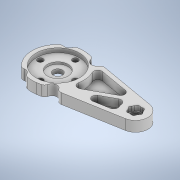
# Autodesk Inventor part: Ankle_side_pitch_frame
Saved by Autodesk Inventor 2020 (Build 240168000, 168)
## iProperties
Created: 2021-10-01
Part Number: Ankle_side_pitch_frame
Material: アルミニウム 2014-T4
Document SubType Name: Modeling
Designer: Masato Kubotera
Density: 2.8 g/cm^3
Appearance: 滑らか - 淡い灰色
Description: A2017 T5
Author: Masato Kubotera
Autodesk Inventor part; units mm, degrees
ref_plane "YZ Plane" through (0, 0, 0) normal (1, 0, 0) x (0, 1, 0)
ref_plane "XZ Plane" through (0, 0, 0) normal (0, 1, 0) x (-1, 0, 0)
ref_plane "XY Plane" through (0, 0, 0) normal (0, 0, 1) x (1, 0, 0)
sketch "スケッチ1" plane through (0, 0, 0) normal (0, 0, 1) x (1, 0, 0)
  circle A0 centre (0, 0) radius 10.5 construction
  circle A1 centre (0, 0) radius 5 construction
  circle A2 centre (0, 0) radius 5.01
  circle A3 centre (0, 0) radius 10.51
  arc A4 (2.1531, 12.3132) -> (2.1531, -12.3132) centre (0, 0) ccw
  circle A5 centre (37.7359, 0) radius 2.25
  arc A6 (38.7694, -5.9103) -> (38.7694, 5.9103) centre (37.7359, 0) ccw
  circle A7 centre (8.5, 0) radius 1.35
  circle A8 centre (0, 8.5) radius 1.35
  circle A9 centre (-8.5, 0) radius 1.35
  circle A10 centre (0, -8.5) radius 1.35
  line L0 (2.1531, 12.3132) -> (38.7694, 5.9103)
  line L1 (2.1531, -12.3132) -> (38.7694, -5.9103)
  line L2 (13.3804, 8.3196) -> (26.7879, 5.9751)
  line L3 (30.7947, -5.2745) -> (23.5904, -6.5342)
  arc A11 (2.1531, -12.3132) -> (-4.7001, 11.5827) centre (0, 0) ccw construction
  arc A12 (38.7694, 5.9103) -> (32.2717, -2.4783) centre (37.7359, 0) ccw construction
  line L4 (34.0196, 4.7105) -> (8.4896, -9.1748) construction
  line L5 (27.399, 2.248) -> (15.2168, -4.3777)
  line L6 (28.8431, 0.7568) -> (22.2903, -2.8072)
  line L7 (32.4358, 4.9875) -> (34.0196, 4.7105) construction
  line L8 (11.5743, -8.6354) -> (8.4896, -9.1748) construction
  arc A13 (31.783, -0.7501) -> (32.2717, -2.4783) centre (37.7359, 0) ccw
  arc A14 (12.2941, -2.2592) -> (11.2378, 5.4737) centre (0, 0) ccw
  line L9 (40.9229, 0) -> (40.3979, -0.9093) construction
  line L10 (39.3294, -2.76) -> (38.2794, -2.76) construction
  line L11 (36.1424, -2.76) -> (35.6174, -1.8507) construction
  line L12 (34.549, 0) -> (35.074, 0.9093) construction
  line L13 (36.1424, 2.76) -> (37.1924, 2.76) construction
  line L14 (39.3294, 2.76) -> (39.8544, 1.8507)
  arc A15 (40.3979, -0.9093) -> (40.3979, 0.9093) centre (39.8729, 0) ccw
  arc A16 (39.8544, 1.8507) -> (38.2794, 2.76) centre (38.8044, 1.8507) ccw
  arc A17 (37.1924, 2.76) -> (35.6174, 1.8507) centre (36.6674, 1.8507) ccw
  arc A18 (35.074, 0.9093) -> (35.074, -0.9093) centre (35.599, 0) ccw
  arc A19 (35.6174, -1.8507) -> (37.1924, -2.76) centre (36.6674, -1.8507) ccw
  arc A20 (38.2794, -2.76) -> (39.8544, -1.8507) centre (38.8044, -1.8507) ccw
  line L15 (40.3979, -0.9093) -> (39.8544, -1.8507)
  line L16 (39.8544, -1.8507) -> (39.3294, -2.76) construction
  line L17 (38.2794, -2.76) -> (37.1924, -2.76)
  line L18 (37.1924, -2.76) -> (36.1424, -2.76) construction
  line L19 (35.6174, -1.8507) -> (35.074, -0.9093)
  line L20 (35.074, -0.9093) -> (34.549, 0) construction
  line L21 (35.6174, 1.8507) -> (36.1424, 2.76) construction
  line L22 (35.074, 0.9093) -> (35.6174, 1.8507)
  line L23 (37.1924, 2.76) -> (38.2794, 2.76)
  line L24 (38.2794, 2.76) -> (39.3294, 2.76) construction
  line L25 (39.8544, 1.8507) -> (40.3979, 0.9093)
  line L26 (40.3979, 0.9093) -> (40.9229, 0) construction
  circle A21 centre (37.7359, 0) radius 1.55
  circle A22 centre (0, 0) radius 2.25
  line L27 (0, 0) -> (27.1359, -16.96) construction
  line L28 (37.7359, 0) -> (27.1359, -16.96) construction
  line L29 (0, 0) -> (37.7359, 0) construction
  line L30 (0, 0) -> (0.848, -0.53)
  line L31 (8.003, 10.918) -> (-6.307, -11.978) construction
  arc A23 (-3.808, -11.9058) -> (-7.6616, -9.8768) centre (-6.307, -11.978) ccw
  arc A24 (5.6301, 11.7052) -> (10.5021, 10.8532) centre (8.003, 10.918) ccw
  arc A25 (13.3804, 8.3196) -> (11.2378, 5.4737) centre (13.0359, 6.3495) ccw
  arc A26 (12.2941, -2.2592) -> (15.2168, -4.3777) centre (14.2612, -2.6207) ccw
  arc A27 (22.2903, -2.8072) -> (23.5904, -6.5342) centre (23.2459, -4.5641) ccw
  arc A28 (30.7947, -5.2745) -> (32.2717, -2.4783) centre (30.4502, -3.3043) ccw
  arc A29 (31.783, -0.7501) -> (28.8431, 0.7568) centre (29.7987, -1.0002) ccw
  arc A30 (27.399, 2.248) -> (26.7879, 5.9751) centre (26.4434, 4.005) ccw
  line L32 (8.003, -10.918) -> (-6.307, 11.978) construction
  arc A31 (-7.6616, 9.8768) -> (-3.808, 11.9058) centre (-6.307, 11.978) ccw
  arc A32 (10.5021, -10.8532) -> (5.6301, -11.7052) centre (8.003, -10.918) ccw
  point P0 (8.4896, 9.1748)
  point P1 (34.0196, -4.7105)
  point P2 (10.3333, -7.0337)
  point P3 (32.3635, 2.6714)
  point P4 (39.3294, 2.76)
  point P5 (9.5861, 8.9831)
  point P6 (9.0332, 8.6401)
  point P7 (-3.808, 11.9058)
  dimension "d0" = 21
  dimension "d1" = 10
  dimension "d2" = 0.01
  dimension "d3" = 0.01
  dimension "d4" = 25
  dimension "d7" = 4.5
  dimension "d8" = 6
  dimension "d9" = 2.7
  dimension "d10" = 8.5
  dimension "d13" = 360
  dimension "d15" = 2
  dimension "d16" = 2
  dimension "d17" = 1
  dimension "d18" = 1
  dimension "d20" = 1.05
  dimension "d23" = 360
  dimension "d25" = 5.52
  dimension "d30" = 3.1
  dimension "d33" = 4.5
  dimension "d41" = 20
  dimension "d42" = 32
  dimension "d46" = 27
  dimension "d47" = 1
  dimension "d48" = 90
  dimension "d49" = 2.5
  dimension "d50" = 2.5
  dimension "d51" = 2
  dimension "d52" = 2
  dimension "d53" = 2
  dimension "d55" = 2.5
  dimension "d56" = 2.5
  constraints: 66 end point, 60 point on circle, 33 centre point, 19 coincident, 16 tangent, 14 point on line, 6 parallel, 3 collinear, 3 equal radius, 2 perpendicular, 2 symmetric about line, 1 horizontal, 1 midpoint, 53 other
  measures "d0" diameter of A0
  measures "d1" diameter of A1
  measures "d2" radial gap between concentric circles of A3 A0
  measures "d3" radial gap between concentric circles of A2 A1
  measures "d4" diameter of A4
  measures "d7" diameter of A5
  measures "d8" radius of A6
  measures "d9" diameter of A7
  measures "d10" distance of point (0, 0) A7.centre
  measures "d15" distance between parallel lines of L0 L2
  measures "d16" distance between parallel lines of L1 L3
  measures "d17" distance between parallel lines of L4 L6
  measures "d18" distance between parallel lines of L5 L4
  measures "d20" radius of A15
  measures "d25" distance between parallel lines of L23 L17
  measures "d30" diameter of A21
  measures "d33" diameter of A22
  measures "d41" distance of L28.start L27.end
  measures "d42" distance of L27.start L27.end
  measures "d46" distance of L31.start L31.end
  measures "d47" distance of L30.start L30.end
  measures "d48" angle of L27 L31
  measures "d49" radius of A23
  measures "d50" radius of A24
  measures "d51" radius of A25
  measures "d52" radius of A28
  measures "d53" radius of A30
  measures "d55" radius of A31
  measures "d56" radius of A32
extrude "押し出し1" add sketch "スケッチ1" along normal blind 5 contours L0 A24 A6 L1 A32 A4 A23 A31
extrude "押し出し2" add sketch "スケッチ1" along normal blind 2.8 contours A16 L14 | L14 L25 A15 L15 A20 L17 A19 L19 A18 L22 A17 L23 A16
extrude "押し出し3" add sketch "スケッチ1" along normal blind 2 contours A5
extrude "押し出し4" add sketch "スケッチ1" along normal blind 3 contours A3
extrude "押し出し5" add sketch "スケッチ1" along normal blind 2 contours A2
extrude "押し出し6" add sketch "スケッチ1" along normal blind 1 contours L2 A30 L5 A26 A14 A25 | L3 A27 L6 A29 A13 A28
fillet "フィレット2" radius 2 8 edges at (-3.808, -11.9058, 2.5) (-7.6616, -9.8768, 2.5) (10.5021, 10.8532, 2.5) (5.6301, 11.7052, 2.5) (5.6301, -11.7052, 2.5) (10.5021, -10.8532, 2.5) (-7.6616, 9.8768, 2.5) (-3.808, 11.9058, 2.5)
equation "\"d3\" = d2"
equation "\"d18\" = d17"
equation "\"d50\" = d49"
